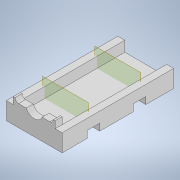
# Autodesk Inventor part: motor_top
Saved by Autodesk Inventor 2020.2 (Build 242310000, 310)
## iProperties
Created: 2020-08-20
Part Number: motor_top
Material: Generic
Document SubType Name: Modeling
Designer: Tarsoly
Density: 1 g/cm^3
Appearance: Default
Author: Tarsoly
Autodesk Inventor part; units mm, degrees
ref_plane "YZ Plane" through (0, 0, 0) normal (1, 0, 0) x (0, 1, 0)
ref_plane "XZ Plane" through (0, 0, 0) normal (0, 1, 0) x (-1, 0, 0)
ref_plane "XY Plane" through (0, 0, 0) normal (0, 0, 1) x (1, 0, 0)
sketch "Sketch1" plane through (0, 0, 0) normal (0, 1, 0) x (-1, 0, 0)
  line L0 (8, 16) -> (-8, 16)
  line L1 (-8, 16) -> (-8, -16)
  line L2 (-8, -16) -> (8, -16)
  line L3 (8, -16) -> (8, 16)
  line L4 (8, 16) -> (-8, -16) construction
  line L5 (-8, 16) -> (8, -16) construction
  point P0 (0, 0)
  dimension "d0" = 16
  dimension "d1" = 32
  constraints: 12 end point, 2 midpoint, 2 parallel, 1 horizontal, 1 perpendicular
  measures "d0" distance of L0.start L0.end
  measures "d1" distance of L2.end L0.start
extrude "Extrusion1" add sketch "Sketch1" along normal blind 2
sketch "Sketch2" plane through (0, 2, 0) normal (0, 1, 0) x (1, 0, 0)
  line L0 (8, 16) -> (-8, 16) projected
  line L1 (-6, 16) -> (6, 16)
  line L2 (6, 16) -> (6, -14)
  line L3 (6, -14) -> (-6, -14)
  line L4 (-6, -14) -> (-6, 16)
  line L5 (8, -16) -> (8, 16) projected
  line L6 (-8, 16) -> (-8, -16) projected
  line L7 (-8, -16) -> (8, -16) projected
  point P0 (0, 0)
  dimension "d4" = 2
  dimension "d5" = 2
  dimension "d6" = 2
  constraints: 8 end point, 2 parallel, 1 horizontal, 1 perpendicular, 1 point on line
  measures "d4" distance between parallel lines of L5 L2
  measures "d5" distance between parallel lines of L6 L4
  measures "d6" distance between parallel lines of L7 L3
extrude "Extrusion2" add sketch "Sketch2" along normal blind 3 contours L5 L7 L6 L0 L4 L3 L2
sketch "Sketch4" plane through (0, 5, 0) normal (0, 1, 0) x (1, 0, 0)
  line L0 (6, -14) -> (-6, -14) projected
  line L1 (-8, -16) -> (8, -16) projected
  line L2 (-6, -14) -> (6, -14)
  line L3 (6, -14) -> (6, -16)
  line L4 (6, -16) -> (-6, -16)
  line L5 (-6, -16) -> (-6, -14)
  line L6 (6, 16) -> (6, -14) projected
  point P0 (0, 0)
  constraints: 8 end point, 2 parallel, 1 collinear, 1 horizontal, 1 perpendicular, 1 point on line
extrude "Extrusion3" add sketch "Sketch4" along normal blind 2
sketch "Sketch3" plane through (-8, 0, 16) normal (0, 0, 1) x (1, 0, 0)
  line L0 (14, 2) -> (2, 2) construction
  line L1 (2, 2) -> (14, 2) construction
  circle A0 centre (8, 7) radius 2.5
  line L2 (8, 11.4) -> (8, -1.9) construction
  line L3 (3.5, 7) -> (12.5, 7) construction
  circle A1 centre (3.5, 7) radius 1
  circle A2 centre (12.5, 7) radius 1
  line L4 (3.5, 8) -> (5.7087, 8)
  line L5 (12.5, 8) -> (10.2913, 8)
  line L6 (12.5, 6) -> (10.2913, 6)
  line L7 (5.7087, 6) -> (3.5, 6)
  point P0 (8, 0)
  dimension "d9" = 5
  dimension "d10" = 5
  dimension "d11" = 9
  dimension "d12" = 2
  dimension "d13" = 2
  constraints: 10 end point, 8 point on circle, 4 point on line, 3 centre point, 3 horizontal, 3 tangent, 2 coincident, 2 midpoint, 1 parallel
  measures "d9" distance from line of L0 A0.centre
  measures "d10" diameter of A0
  measures "d11" distance of L3.start L3.end
  measures "d12" diameter of A2
  measures "d13" diameter of A1
extrude "Extrusion4" cut sketch "Sketch3" against normal up to next
ref_plane "Work Plane1" through (6, 2, 7) normal (0, 0, -1) x (-1, 0, 0)
ref_plane "Work Plane2" through (6, 2, -8) normal (0, 0, -1) x (-1, 0, 0)
sketch "Sketch6" plane through (6, 2, 7) normal (0, 0, -1) x (-1, 0, 0)
  line L0 (-2, -2) -> (-2, 0)
  line L1 (-2, -2) -> (-2, 3) projected
  line L2 (-2, 0) -> (0, -2)
  line L3 (-2, -2) -> (14, -2) projected
  line L4 (0, -2) -> (-2, -2)
  line L5 (6, -3.4) -> (6, 6.4) construction
  line L6 (14, -2) -> (14, 0)
  line L7 (14, 0) -> (12, -2)
  line L8 (12, -2) -> (14, -2)
  point P0 (6, -2)
  dimension "d22" = 2
  dimension "d23" = 45
  constraints: 12 end point, 2 point on line, 2 symmetric about line, 1 collinear
  measures "d22" distance of L0.start L0.end
  measures "d23" angle of L0 L2
extrude "Extrusion5" cut sketch "Sketch6" along normal mid plane 3.6
sketch "Sketch7" plane through (6, 2, -8) normal (0, 0, -1) x (-1, 0, 0)
  line L0 (-2, 0) -> (0, -2) projected
  line L1 (-2, -2) -> (-2, 0) projected
  line L2 (0, -2) -> (-2, -2) projected
  line L3 (12, -2) -> (14, 0) projected
  line L4 (14, -2) -> (12, -2) projected
  line L5 (14, 0) -> (14, -2) projected
  point P0 (6, -2)
extrude "Extrusion6" cut sketch "Sketch7" against normal blind 3.6
equation "\"d5\" = d4"
equation "\"d6\" = d4"
body "Solid1"
